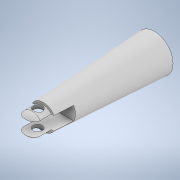
# Autodesk Inventor part: arms
Saved by Autodesk Inventor 2021 (Build 250183000, 183)
## iProperties
Created: 2021-06-26
Part Number: arms
Material: Generic
Document SubType Name: Modeling
Designer: TARUN
Density: 1 g/cm^3
Appearance: Default
Author: TARUN
Autodesk Inventor part; units mm, degrees
ref_plane "YZ Plane" through (0, 0, 0) normal (1, 0, 0) x (0, 1, 0)
ref_plane "XZ Plane" through (0, 0, 0) normal (0, 1, 0) x (-1, 0, 0)
ref_plane "XY Plane" through (0, 0, 0) normal (0, 0, 1) x (1, 0, 0)
sketch "Sketch1" plane through (0, 0, 0) normal (0, 0, 1) x (1, 0, 0)
  circle A0 centre (0, 0) radius 5
  dimension "d0" = 10
  constraints: 1 centre point, 1 coincident
  measures "d0" diameter of A0
extrude "Extrusion1" add sketch "Sketch1" along normal blind 30 draft -3
sketch "Sketch2" plane through (0, 0, 30) normal (0, 0, 1) x (1, 0, 0)
  circle A0 centre (0, 0) radius 2.8754
  constraints: 1 centre point, 1 coincident
extrude "Extrusion2" add sketch "Sketch2" along normal blind 5
fillet "Fillet1" radius 2 1 edges at (-2.8754, 0, 35)
sketch "Sketch4" plane through (0, 0, 0) normal (0, 1, 0) x (-1, 0, 0)
  circle A0 centre (0, 31.4792) radius 1.25
  point P0 (0, 0)
  dimension "d8" = 2.5
  constraints: 1 centre point
  measures "d8" diameter of A0
extrude "Extrusion4" cut sketch "Sketch4" along normal mid plane 10
sketch "Sketch5" plane through (0, 0, 35) normal (0, 0, 1) x (1, 0, 0)
  circle A0 centre (0, 0) radius 5 projected
  line L0 (-4.6538, 1.8283) -> (4.6538, 1.8283)
  line L1 (4.6538, -1.8283) -> (-4.6538, -1.8283)
  arc A1 (-4.6538, 1.8283) -> (-4.6538, -1.8283) centre (0, 0) ccw
  arc A2 (4.6538, -1.8283) -> (4.6538, 1.8283) centre (0, 0) ccw
  constraints: 8 point on circle, 4 end point, 2 centre point, 2 concentric, 1 horizontal, 1 parallel
extrude "Extrusion5" cut sketch "Sketch5" against normal blind 10 contours A0 L1 L0
body "Solid1"
